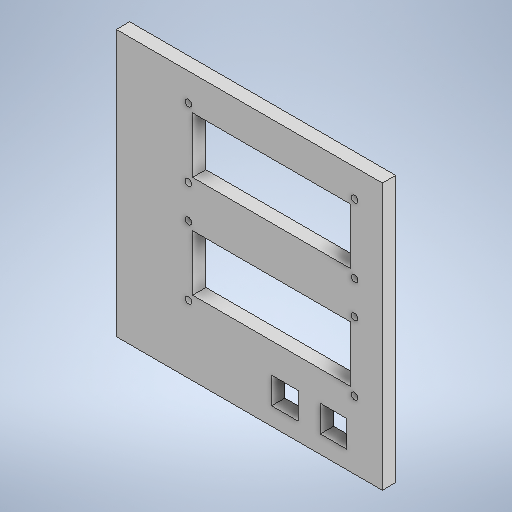
# Autodesk Inventor part: lcd holder
Saved by Autodesk Inventor 2025.3 (Build 293356000, 356)
## iProperties
Created: 2026-05-01
Part Number: lcd holder
Material: Generic
Document SubType Name: Modeling
Designer: kamal
Density: 1 g/cm^3
Appearance: Default
Author: kamal
Autodesk Inventor part; units mm, degrees
ref_plane "YZ Plane" through (0, 0, 0) normal (1, 0, 0) x (0, 1, 0)
ref_plane "XZ Plane" through (0, 0, 0) normal (0, 1, 0) x (-1, 0, 0)
ref_plane "XY Plane" through (0, 0, 0) normal (0, 0, 1) x (1, 0, 0)
sketch "Sketch1" plane through (0, 0, 0) normal (0, 0, 1) x (1, 0, 0)
  line L0 (0, 0) -> (200, 0)
  line L1 (200, 0) -> (200, 120)
  line L2 (200, 120) -> (0, 120)
  line L3 (0, 120) -> (0, 0)
  line L4 (110, 110) -> (190, 110) construction
  line L5 (190, 110) -> (190, 74) construction
  line L6 (190, 74) -> (110, 74) construction
  line L7 (110, 74) -> (110, 110) construction
  line L8 (110, 64) -> (190, 64) construction
  line L9 (190, 64) -> (190, 28) construction
  line L10 (190, 28) -> (110, 28) construction
  line L11 (110, 28) -> (110, 64) construction
  circle A0 centre (112.5, 107.5) radius 1.5
  circle A1 centre (112.5, 61.5) radius 1.5
  circle A2 centre (187.5, 61.5) radius 1.5
  circle A3 centre (112.5, 30.5) radius 1.5
  circle A4 centre (187.5, 30.5) radius 1.5
  circle A5 centre (187.5, 107.5) radius 1.5
  circle A6 centre (112.5, 76.5) radius 1.5
  circle A7 centre (187.5, 76.5) radius 1.5
  line L12 (114.4, 104.6) -> (185.6, 104.6)
  line L13 (185.6, 104.6) -> (185.6, 79.4)
  line L14 (185.6, 79.4) -> (114.4, 79.4)
  line L15 (114.4, 79.4) -> (114.4, 104.6)
  line L16 (114.4, 58.6) -> (185.6, 58.6)
  line L17 (185.6, 58.6) -> (185.6, 33.4)
  line L18 (185.6, 33.4) -> (114.4, 33.4)
  line L19 (114.4, 33.4) -> (114.4, 58.6)
  dimension "d0" = 200
  dimension "d1" = 120
  dimension "d4" = 80
  dimension "d5" = 36
  dimension "d6" = 80
  dimension "d7" = 36
  dimension "d8" = 110
  dimension "d9" = 110
  dimension "d10" = 10
  dimension "d11" = 10
  dimension "d12" = 3
  dimension "d13" = 2.5
  dimension "d14" = 2.5
  dimension "d15" = 3
  dimension "d16" = 2.5
  dimension "d17" = 2.5
  dimension "d20" = 75
  dimension "d23" = 31
  dimension "d28" = 75
  dimension "d31" = 31
  dimension "d34" = 5.4
  dimension "d35" = 4.4
  dimension "d36" = 4.4
  dimension "d37" = 5.4
  dimension "d38" = 5.4
  dimension "d39" = 4.4
  dimension "d40" = 5.4
  dimension "d41" = 4.4
  constraints: 40 end point, 10 parallel, 8 centre point, 7 horizontal, 5 perpendicular, 2 vertical, 12 other
  measures "d0" distance of L2.end L1.end
  measures "d1" distance of L0.end L1.end
  measures "d4" distance of L5.end L6.end
  measures "d5" distance of L4.end L5.end
  measures "d6" distance of L9.end L10.end
  measures "d7" distance of L8.end L9.end
  measures "d8" distance between parallel lines of L3 L7
  measures "d9" distance between parallel lines of L3 L11
  measures "d10" distance between parallel lines of L4 L2
  measures "d11" distance between parallel lines of L8 L6
  measures "d12" diameter of A0
  measures "d13" distance from line of A0.centre L4
  measures "d14" distance from line of L7 A0.centre
  measures "d15" diameter of A1
  measures "d16" distance from line of L8 A1.centre
  measures "d17" distance from line of L11 A1.centre
  measures "d20" distance of A1.centre A2.centre
  measures "d23" distance of A1.centre A3.centre
  measures "d28" distance of A0.centre A5.centre
  measures "d31" distance of A0.centre A6.centre
  measures "d34" distance between parallel lines of L4 L12
  measures "d35" distance between parallel lines of L7 L15
  measures "d36" distance between parallel lines of L5 L13
  measures "d37" distance between parallel lines of L6 L14
  measures "d38" distance between parallel lines of L8 L16
  measures "d39" distance between parallel lines of L11 L19
  measures "d40" distance between parallel lines of L10 L18
  measures "d41" distance between parallel lines of L9 L17
extrude "Extrusion1" add sketch "Sketch1" along normal blind 6
extrude "Extrusion2" cut sketch "Sketch1" along normal blind 75 contours A0 | A1 | A2 | A3 | A4 | A5 | A6 | A7 | L12 L13 L14 L15 | L16 L17 L18 L19
sketch "Sketch2" plane through (0, 0, 0) normal (0, 0, -1) x (-1, 0, 0)
  line L0 (-150, 8) -> (-162, 8)
  line L1 (-162, 8) -> (-162, 20)
  line L2 (-162, 20) -> (-150, 20)
  line L3 (-150, 20) -> (-150, 8)
  line L4 (-172, 8) -> (-184, 8)
  line L5 (-184, 8) -> (-184, 20)
  line L6 (-184, 20) -> (-172, 20)
  line L7 (-172, 20) -> (-172, 8)
  line L8 (0, 120) -> (0, 0) projected
  line L9 (-200, 120) -> (0, 120) projected
  point P0 (-150, 14)
  point P1 (-172, 14)
  dimension "d44" = 12
  dimension "d45" = 12
  dimension "d46" = 12
  dimension "d47" = 12
  dimension "d48" = 150
  dimension "d49" = 10
  dimension "d50" = 100
  dimension "d51" = 100
  constraints: 16 end point, 4 parallel, 2 horizontal, 2 midpoint, 2 perpendicular
  measures "d44" distance of L1.end L2.end
  measures "d45" distance of L0.end L1.end
  measures "d46" distance of L5.end L6.end
  measures "d47" distance of L4.end L5.end
  measures "d48" distance from line of L8 point (-150, 14)
  measures "d49" distance from line of point (-172, 14) L1
  measures "d50" distance between parallel lines of L9 L2
  measures "d51" distance between parallel lines of L9 L6
extrude "Extrusion3" cut sketch "Sketch2" against normal blind 6
sketch "Sketch3" plane through (0, 0, 6) normal (0, 0, 1) x (1, 0, 0)
  line L0 (0, 0) -> (200, 0) projected
  line L1 (0, 120) -> (80, 120)
  line L2 (80, 120) -> (80, 0)
  line L3 (80, 0) -> (0, 0)
  line L4 (0, 0) -> (0, 120)
  dimension "d54" = 80
  constraints: 8 end point, 2 parallel, 1 horizontal, 1 perpendicular, 1 point on line
  measures "d54" distance of L2.end L3.end
extrude "Extrusion4" cut sketch "Sketch3" against normal blind 10
equation "\"d42\" = d28"
body "Solid1"
